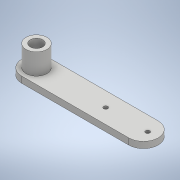
# Autodesk Inventor part: элемент-2
Saved by Autodesk Inventor 2020 (Build 240168000, 168)
## iProperties
Created: 2020-01-23
Part Number: элемент-2
Material: Типовые
Document SubType Name: Modeling
Designer: Css38
Density: 1 g/cm^3
Appearance: По умолчанию
Author: Css38
Autodesk Inventor part; units mm, degrees
ref_plane "YZ Plane" through (0, 0, 0) normal (1, 0, 0) x (0, 1, 0)
ref_plane "XZ Plane" through (0, 0, 0) normal (0, 1, 0) x (-1, 0, 0)
ref_plane "XY Plane" through (0, 0, 0) normal (0, 0, 1) x (1, 0, 0)
sketch "Эскиз1" plane through (0, 0, 0) normal (0, 0, 1) x (1, 0, 0)
  line L0 (0, 0) -> (25.5, 0) construction
  line L1 (0, -3.5) -> (25.5, -3.5)
  line L2 (25.5, 3.5) -> (0, 3.5)
  arc A0 (0, 3.5) -> (0, -3.5) centre (0, 0) ccw
  arc A1 (25.5, -3.5) -> (25.5, 3.5) centre (25.5, 0) ccw
  point P0 (12.75, 0)
  dimension "d0" = 25.5
  dimension "d1" = 7
  constraints: 8 end point, 4 point on circle, 4 tangent, 2 centre point, 1 horizontal, 1 midpoint, 1 parallel
  measures "d0" distance of L0.start L0.end
  measures "d1" diameter of A1
extrude "Выдавливание1" add sketch "Эскиз1" along normal blind 1.5
sketch "Эскиз2" plane through (0, 0, 1.5) normal (0, 0, 1) x (1, 0, 0)
  circle A0 centre (0, 0) radius 2.5
  circle A1 centre (0, 0) radius 1.5
  dimension "d4" = 5
  dimension "d5" = 1
  constraints: 2 centre point, 1 coincident
  measures "d4" diameter of A0
  measures "d5" radial gap between concentric circles of A0 A1
extrude "Выдавливание2" add sketch "Эскиз2" along normal blind 5
sketch "Эскиз6" plane through (0, 0, 0) normal (0, 0, 1) x (1, 0, 0)
  line L0 (-10, 0) -> (35.5, 0) construction
  arc A0 (25.5, -3.5) -> (25.5, 3.5) centre (25.5, 0) ccw construction
  circle A1 centre (26.5, 0) radius 0.5
  circle A2 centre (16.5, 0) radius 0.5
  point P0 (0, 0)
  point P1 (29, 0)
  point P2 (29, 0)
  dimension "d22" = 1
  dimension "d23" = 2.5
  dimension "d25" = 10
  constraints: 3 point on line, 2 centre point, 2 point on circle, 1 equal radius
  measures "d22" diameter of A1
  measures "d23" distance of point (29, 0) A1.centre
  measures "d25" distance of A2.centre A1.centre
hole "Отверстие1" at (26.5, 0, 0) at (16.5, 0, 0) direction (0, 0, 1) diameter 1 end through all countersink diameter 1.5 countersink angle 90
